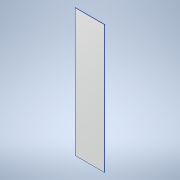
# Autodesk Inventor part: 7000_Aluminum_Chasis_Coil_Assembly_Separator_MPSv2_v1
Saved by Autodesk Inventor 2021 (Build 250183000, 183)
## iProperties
Created: 2020-11-18
Part Number: 7000_Aluminum_Chasis_Coil_Assembly_Separator_MPSv2_v1
Material: Aluminum 6061
Document SubType Name: Modeling
Designer: Admin
Density: 2.7 g/cm^3
Appearance: Aluminum - Flat
Author: Admin
Autodesk Inventor part; units mm, degrees
ref_plane "YZ Plane" through (0, 0, 0) normal (1, 0, 0) x (0, 1, 0)
ref_plane "XZ Plane" through (0, 0, 0) normal (0, 1, 0) x (-1, 0, 0)
ref_plane "XY Plane" through (0, 0, 0) normal (0, 0, 1) x (1, 0, 0)
sketch "Sketch1" plane through (0, 0, 0) normal (0, 0, 1) x (1, 0, 0)
  line L0 (0, 0) -> (97.693, 0)
  line L1 (97.693, 0) -> (97.693, -427.888)
  line L2 (97.693, -427.888) -> (0, -427.888)
  line L3 (0, -427.888) -> (0, 0)
  dimension "d0" = 97.693
  dimension "d1" = 427.888
  constraints: 8 end point, 2 parallel, 1 horizontal, 1 perpendicular
  measures "d0" distance of L1.end L2.end
  measures "d1" distance of L0.end L1.end
extrude "Extrusion1" add sketch "Sketch1" along normal blind 1.295
body "Solid1"
